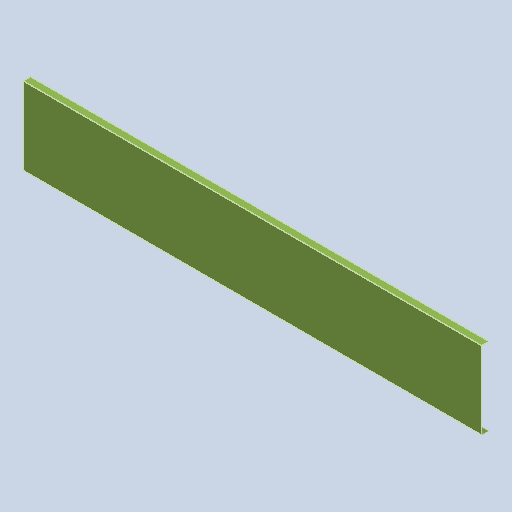
# Autodesk Inventor part: Acoplador_de_Cuentas
Saved by Autodesk Inventor 2023 (Build 270158000, 158)
## iProperties
Created: 2022-11-09
Part Number: Acoplador_de_Cuentas
Material: Generic
Document SubType Name: Sheet Metal
Designer: David
Density: 1 g/cm^3
Sheet Metal Rule: Default_mm
Appearance: Olive Green
Author: David
Autodesk Inventor part; units mm, degrees
ref_plane "YZ Plane" through (0, 0, 0) normal (1, 0, 0) x (0, 1, 0)
ref_plane "XZ Plane" through (0, 0, 0) normal (0, 1, 0) x (-1, 0, 0)
ref_plane "XY Plane" through (0, 0, 0) normal (0, 0, 1) x (1, 0, 0)
sketch "Sketch1" plane through (0, 0, 0) normal (0, 0, 1) x (1, 0, 0)
  line L0 (-796.5, -135) -> (796.5, -135)
  line L1 (796.5, -135) -> (796.5, 135)
  line L2 (796.5, 135) -> (-796.5, 135)
  line L3 (-796.5, 135) -> (-796.5, -135)
  line L4 (-796.5, -135) -> (796.5, 135) construction
  line L5 (796.5, -135) -> (-796.5, 135) construction
  point P0 (0, 0)
  dimension "d0" = 1593
  dimension "d1" = 270
  measures "d0" distance of L2.end L1.end
  measures "d1" distance of L1.end L0.end
extrude "Plate1" add sketch "Sketch1" along normal blind 0.5
sketch "Sketch2" plane through (796.5, 134.5, 0.5) normal (0, 1, 0) x (-1, 0, 0)
  line L0 (1593, 0) -> (0, 0)
  line L1 (0, 0) -> (0, -25)
  line L2 (0, -25) -> (1593, -25)
  line L3 (1593, -25) -> (1593, 0)
  constraints: 6 end point, 1 horizontal, 1 perpendicular, 1 vertical
edge flange "Flange1" height 25 angle 90 thickness 0.5 bend radius 0.5 thickness toward (0, 1, 0) relief straight relief width 0.5 relief depth 0.25 corner gap 0.5 corner form 0 edges at (0, 135, 0) (0, -135, 0) wall of the first edge with corners at (-796.5, 134.5, 0.5) (796.5, 134.5, 0.5) (796.5, 134.5, -24.5) (-796.5, 134.5, -24.5)
bend "Bend1"
corner "Corner1"
equation "\"d2\" = Thickness"
equation "\"d3\" = BendReliefWidth"
equation "\"d4\" = BendReliefDepth"
equation "\"d5\" = MinimumRemnant"
equation "\"d6\" = TransitionRadius"
equation "\"d9\" = BendRadius"
equation "\"d10\" = CornerReliefSize"
equation "\"d11\" = GapSize"
equation "\"d12\" = JacobiRadiusSize"
equation "\"BendRadius\" = Thickness"
equation "\"BendReliefWidth\" = Thickness"
equation "\"BendReliefDepth\" = 0.5 * Thickness"
equation "\"CornerReliefSize\" = 4 * Thickness"
equation "\"MinimumRemnant\" = 2 * Thickness"
equation "\"TransitionRadius\" = BendRadius"
equation "\"JacobiRadiusSize\" = BendRadius"
equation "\"GapSize\" = Thickness"
equation "\"Space7\" = 0"
equation "\"Thickness\" = 0.5"
body "Solid1"
